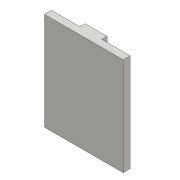
# Autodesk Inventor part: BMS
Saved by Autodesk Inventor 2018 (Build 220112000, 112)
## iProperties
Created: 2019-09-10
Part Number: BMS
Material: Generic
Document SubType Name: Modeling
Designer: Clevo
Density: 1 g/cm^3
Appearance: Default
Author: Clevo
Autodesk Inventor part; units mm, degrees
ref_plane "YZ Plane" through (0, 0, 0) normal (1, 0, 0) x (0, 1, 0)
ref_plane "XZ Plane" through (0, 0, 0) normal (0, 1, 0) x (-1, 0, 0)
ref_plane "XY Plane" through (0, 0, 0) normal (0, 0, 1) x (1, 0, 0)
sketch "Sketch1" plane through (0, 0, 0) normal (0, 1, 0) x (-1, 0, 0)
  line L0 (-22.5, -28) -> (22.5, -28)
  line L1 (22.5, -28) -> (22.5, 28)
  line L2 (22.5, 28) -> (-22.5, 28)
  line L3 (-22.5, 28) -> (-22.5, -28)
  line L4 (-22.5, -28) -> (22.5, 28) construction
  line L5 (22.5, -28) -> (-22.5, 28) construction
  point P0 (0, 0)
  dimension "d0" = 56
  dimension "d1" = 45
  constraints: 12 end point, 2 midpoint, 2 parallel, 1 horizontal, 1 perpendicular
  measures "d0" distance of L0.end L1.end
  measures "d1" distance of L1.end L2.end
extrude "Extrusion1" add sketch "Sketch1" along normal blind 4
sketch "Sketch2" plane through (0, 4, 0) normal (0, 1, 0) x (1, 0, 0)
  line L0 (-6.25, -28) -> (6.25, -28)
  line L1 (6.25, -28) -> (6.25, -18)
  line L2 (6.25, -18) -> (-6.25, -18)
  line L3 (-6.25, -18) -> (-6.25, -28)
  line L4 (-22.5, -28) -> (22.5, -28) projected
  point P0 (0, 0)
  point P1 (0, -18)
  dimension "d4" = 12.5
  dimension "d5" = 10
  constraints: 8 end point, 2 parallel, 1 collinear, 1 horizontal, 1 midpoint, 1 perpendicular, 1 vertical alignment
  measures "d4" distance of L1.end L2.end
  measures "d5" distance of L2.end L0.start
extrude "Extrusion2" add sketch "Sketch2" along normal blind 3
body "Solid1"
